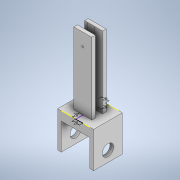
# Autodesk Inventor part: S.Platform
Saved by Autodesk Inventor 2020 (Build 240168000, 168)
## iProperties
Created: 2020-04-14
Part Number: S.Platform
Material: Generic
Document SubType Name: Modeling
Designer: Darugar
Density: 1 g/cm^3
Appearance: Default
Author: Darugar
Autodesk Inventor part; units mm, degrees
ref_plane "YZ Plane" through (0, 0, 0) normal (1, 0, 0) x (0, 1, 0)
ref_plane "XZ Plane" through (0, 0, 0) normal (0, 1, 0) x (-1, 0, 0)
ref_plane "XY Plane" through (0, 0, 0) normal (0, 0, 1) x (1, 0, 0)
sketch "Sketch1" plane through (0, 0, 0) normal (0, 0, 1) x (1, 0, 0)
  line L0 (0, 0) -> (100, 0)
  line L1 (100, 0) -> (100, 100)
  line L2 (100, 100) -> (0, 100)
  line L3 (0, 100) -> (0, 0)
  dimension "d0" = 100
  dimension "d1" = 100
  constraints: 8 end point, 2 parallel, 1 horizontal, 1 perpendicular
  measures "d0" distance of L2.end L1.end
  measures "d1" distance of L1.end L0.end
extrude "Extrusion1" add sketch "Sketch1" along normal blind 80
sketch "Sketch2" plane through (0, 0, 80) normal (0, 0, 1) x (1, 0, 0)
  line L0 (0, 100) -> (0, 0) projected
  line L1 (0, 50) -> (10, 50)
  line L2 (100, 100) -> (0, 100) projected
  line L3 (50, 100) -> (50, 75)
  line L4 (100, 0) -> (100, 100) projected
  line L5 (100, 53.1095) -> (100, 43.1095)
  line L6 (100, 43.1095) -> (90, 43.1095)
  line L7 (0, 0) -> (100, 0) projected
  line L8 (10, 75) -> (90, 75)
  line L9 (90, 75) -> (90, 0)
  line L10 (90, 0) -> (10, 0)
  line L11 (10, 0) -> (10, 75)
  dimension "d4" = 10
  dimension "d5" = 25
  dimension "d6" = 10
  dimension "d7" = 10
  constraints: 16 end point, 3 point on line, 2 horizontal, 2 midpoint, 2 parallel, 2 perpendicular, 1 vertical
  measures "d4" distance of L1.start L1.end
  measures "d5" distance of L3.start L3.end
  measures "d6" distance of L5.start L5.end
  measures "d7" distance of L5.end L6.end
extrude "Extrusion2" cut sketch "Sketch2" against normal blind 80 contours L11 L8 L9 L7
sketch "Sketch3" plane through (0, 100, 0) normal (0, 1, 0) x (1, 0, 0)
  line L0 (90, 0) -> (10, 0) projected
  line L1 (32.4733, 0) -> (52.4733, 0)
  line L2 (52.4733, 0) -> (52.4733, -20)
  line L3 (10, -80) -> (90, -80) projected
  line L4 (70.0717, -80) -> (50.0717, -80)
  line L5 (50.0717, -80) -> (50.0717, -60)
  point P0 (0, 0)
  dimension "d10" = 20
  dimension "d11" = 20
  dimension "d12" = 20
  dimension "d13" = 20
  constraints: 8 end point, 4 point on line, 2 perpendicular
  measures "d10" distance of L1.start L1.end
  measures "d11" distance of L1.end L2.end
  measures "d12" distance of L4.start L4.end
  measures "d13" distance of L4.end L5.end
sketch "Sketch4" plane through (0, 100, 0) normal (0, 1, 0) x (1, 0, 0)
  line L0 (0, 0) -> (0, -80) projected
  line L1 (0, -49.1237) -> (0, -24.1237)
  line L2 (0, -24.1237) -> (25, -24.1237)
  line L3 (100, 0) -> (100, -80) projected
  line L4 (100, -53.0628) -> (100, -28.0628)
  line L5 (100, -28.0628) -> (75, -28.0628)
  line L6 (25, -20.093) -> (75, -20.093)
  line L7 (75, -20.093) -> (75, -30.093)
  line L8 (75, -30.093) -> (25, -30.093)
  line L9 (25, -30.093) -> (25, -20.093)
  line L10 (33.3829, -30.093) -> (33.3829, -30.0462)
  line L11 (33.3829, -30.0462) -> (53.3829, -30.0462)
  line L12 (53.3829, -30.0462) -> (53.3829, -50.0462)
  line L13 (25, -50.0462) -> (75, -50.0462)
  line L14 (75, -50.0462) -> (75, -60.0462)
  line L15 (75, -60.0462) -> (25, -60.0462)
  line L16 (25, -60.0462) -> (25, -50.0462)
  point P0 (53.3829, -30.093)
  dimension "d14" = 25
  dimension "d15" = 25
  dimension "d16" = 90
  dimension "d18" = 25
  dimension "d19" = 90
  dimension "d20" = 50
  dimension "d21" = 10
  dimension "d22" = 20
  dimension "d23" = 20
  dimension "d24" = 50
  dimension "d25" = 10
  constraints: 30 end point, 7 perpendicular, 4 parallel, 4 point on line, 2 horizontal, 1 collinear
  measures "d14" distance of L1.start L1.end
  measures "d15" distance of L1.end L2.end
  measures "d16" angle of L1 L2
  measures "d18" distance of L4.end L5.end
  measures "d19" angle of L5 L4
  measures "d20" distance of L7.end L8.end
  measures "d21" distance of L6.end L7.end
  measures "d22" distance of L10.end L11.end
  measures "d23" distance of L11.end L12.end
  measures "d24" distance of L14.end L15.end
  measures "d25" distance of L13.end L14.end
extrude "Extrusion3" add sketch "Sketch4" along normal blind 200 contours L13 L14 L15 L16 | L6 L7 L8 L12 L11 L10 L9
sketch "Sketch5" plane through (75, 100, 20.093) normal (0, 0, -1) x (-1, 0, 0)
  point P0 (75, -100)
sketch "Sketch6" plane through (75, 100, 20.093) normal (0, 0, -1) x (-1, 0, 0)
  line L0 (0, 0) -> (0, 200) projected
  line L1 (0, 200) -> (25, 200)
  line L2 (21.6171, 200) -> (0, 200) projected
  line L3 (25, 200) -> (25, 165)
  circle A0 centre (25, 165) radius 2.5
  point P0 (75, -100)
  dimension "d28" = 25
  dimension "d29" = 35
  dimension "d30" = 5
  constraints: 4 end point, 1 centre point, 1 coincident, 1 collinear, 1 perpendicular
  measures "d28" distance of L0.end L1.end
  measures "d29" distance of L1.end L3.end
  measures "d30" diameter of A0
extrude "Extrusion4" cut sketch "Sketch6" against normal blind 200
sketch "Sketch7" plane through (100, 0, 0) normal (1, 0, 0) x (0, 0, -1)
  line L0 (0, 0) -> (-80, 0) projected
  line L1 (-40, 0) -> (-40, 14)
  line L2 (-40, 0) -> (-40, 29.8709)
  line L3 (-39.9627, -1.129) -> (-39.9627, 29.871)
  circle A0 centre (-39.9627, 29.871) radius 15.8
  dimension "d33" = 14
  dimension "d34" = 31
  dimension "d35" = 31
  dimension "d36" = 31.6
  constraints: 6 end point, 1 centre point, 1 coincident, 1 midpoint, 1 vertical
  measures "d33" distance of L1.start L1.end
  measures "d34" distance of L2.end L3.start
  measures "d35" distance of L3.start L3.end
  measures "d36" diameter of A0
extrude "Extrusion5" cut sketch "Sketch7" against normal blind 200 contours A0
body "Solid1"
